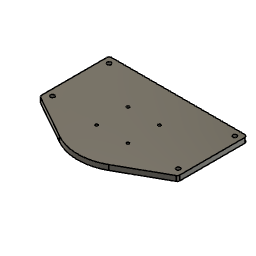
move_base_gnss_plate (Autodesk Fusion 360 design; units mm, degrees)
Autodesk Fusion 360 part; units mm, degrees
note: some values were not read from the file. Set by a fixed rule: the direction of a hole.
sketch "スケッチ1" plane through (0, 0, 0) normal (0, 1, 0) x (1, 0, 0)
  circle A0 centre (0, 0) radius 40
  line L0 (-50, -10) -> (50, -10)
  line L1 (50, -10) -> (50, 35)
  line L2 (50, 35) -> (-50, 35)
  line L3 (-50, 35) -> (-50, -10)
  line L4 (-55, -15) -> (55, -15)
  line L5 (55, -15) -> (55, 40)
  line L6 (55, 40) -> (-55, 40)
  line L7 (-55, 40) -> (-55, -15)
  line L8 (-55, -15) -> (-19.5778, -34.8814)
  line L9 (55, -15) -> (19.5778, -34.8814)
  line L10 (12.5, 12.5) -> (-12.5, 12.5)
  line L11 (-12.5, 12.5) -> (-12.5, -12.5)
  line L12 (-12.5, -12.5) -> (12.5, -12.5)
  line L13 (12.5, -12.5) -> (12.5, 12.5)
  line L14 (12.5, 12.5) -> (-12.5, -12.5) construction
  line L15 (-12.5, 12.5) -> (12.5, -12.5) construction
  point P0 (0, -10)
  dimension "d1" = 80
  dimension "d2" = 100
  dimension "d3" = 10
  dimension "d4" = 35
  dimension "d5" = 5
  dimension "d6" = 5
  dimension "d7" = 5
  dimension "d15" = 25
  constraint coincident A0.centre origin
  constraint horizontal L0
  constraint vertical L1
  constraint horizontal L2
  constraint vertical L3
  constraint midpoint L0 P0
  constraint vertical A0.centre P0
  constraint horizontal L4
  constraint vertical L5
  constraint horizontal L6
  constraint vertical L7
  constraint tangent A0 L6
  constraint coincident A0 L8.end
  constraint coincident A0 L9.end
  constraint tangent A0 L9
  constraint tangent A0 L8
  constraint horizontal L10
  constraint perpendicular L10 L11
  constraint parallel L10 L12
  constraint parallel L11 L13
  constraint coincident L14 A0.centre
  constraint coincident L15 A0.centre
  constraint equal L10 L11
  measures "d1" diameter of A0
  measures "d2" distance of L0.start L0.end
  measures "d3" distance of A0.centre L0
  measures "d4" distance of A0.centre L2
  measures "d5" distance of L1 L5
  measures "d6" distance of L3 L7
  measures "d7" distance of L0 L4
  measures "d15" distance of L10.start L10.end
extrude "押し出し1" add sketch "スケッチ1" along normal blind 4
hole "穴1" at (-50, 0, 10) at (-50, 0, -35) at (50, 0, -35) at (50, 0, 10) direction (0, 1, 0) diameter 3.2 end through all
fillet "フィレット1" radius 2 4 edges at (-55, 2, 15) (-55, 2, -40) (55, 2, 15) (55, 2, -40)
hole "穴2" at (-12.5, 0, 12.5) at (12.5, 0, 12.5) at (12.5, 0, -12.5) at (-12.5, 0, -12.5) direction (0, 1, 0) diameter 2.1 end through all
